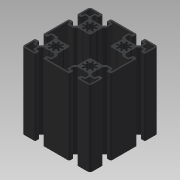
# Autodesk Inventor part: 45-9090
Saved by Autodesk Inventor 2013 (Build 170138000, 138)
## iProperties
Company: 80/20 Inc.
Created: 2014-04-23
Part Number: 45-9090
Material: Generic
Document SubType Name: Modeling
Designer: Ross Bowman
Density: 1 g/cm^3
Engineer: Ross Bowman
Catalog Web Link: 8020.net
Vendor: 80/20 Inc.
Material: 6105-T5 Aluminum
Author: Ross Bowman
Keywords: 80/20 , 8020 , T-Slot , Extrusion
Autodesk Inventor part; units mm, degrees
ref_plane "YZ Plane" through (0, 0, 0) normal (1, 0, 0) x (0, 1, 0)
ref_plane "XZ Plane" through (0, 0, 0) normal (0, 1, 0) x (-1, 0, 0)
ref_plane "XY Plane" through (0, 0, 0) normal (0, 0, 1) x (1, 0, 0)
sketch "Sketch1" plane through (0, 0, 0) normal (0, 0, 1) x (1, 0, 0)
  arc A0 (-37.7086, -41.7083) -> (-39.157, -41.2762) centre (-38.62, -42.1198) ccw
  arc A1 (-37.5167, -42.1716) -> (-37.7086, -41.7083) centre (-45, -45) ccw
  arc A2 (-38.2355, -43.5014) -> (-37.5167, -42.1716) centre (-38.4521, -42.5251) ccw
  line L0 (-38.2355, -43.5014) -> (-40.1182, -43.9192)
  arc A3 (-40.1181, -46.0805) -> (-40.1182, -43.9192) centre (-45, -45) ccw
  line L1 (-40.1181, -46.0805) -> (-38.2353, -46.4985)
  arc A4 (-37.5166, -47.8283) -> (-38.2353, -46.4985) centre (-38.452, -47.4747) ccw
  arc A5 (-37.7085, -48.2915) -> (-37.5166, -47.8283) centre (-45, -45) ccw
  arc A6 (-39.1571, -48.7236) -> (-37.7085, -48.2915) centre (-38.6199, -47.8801) ccw
  line L2 (-39.1571, -48.7236) -> (-40.7838, -47.6877)
  arc A7 (-42.312, -49.216) -> (-40.7838, -47.6877) centre (-45, -45) ccw
  line L3 (-42.312, -49.216) -> (-41.2762, -50.843)
  arc A8 (-41.7083, -52.2914) -> (-41.2762, -50.843) centre (-42.1198, -51.38) ccw
  arc A9 (-42.1716, -52.4833) -> (-41.7083, -52.2914) centre (-45, -45) ccw
  arc A10 (-43.5014, -51.7645) -> (-42.1716, -52.4833) centre (-42.5251, -51.5479) ccw
  line L4 (-43.5014, -51.7645) -> (-43.9192, -49.8818)
  arc A11 (-46.0805, -49.8819) -> (-43.9192, -49.8818) centre (-45, -45) ccw
  line L5 (-46.0805, -49.8819) -> (-46.4985, -51.7647)
  arc A12 (-47.8283, -52.4834) -> (-46.4985, -51.7647) centre (-47.4747, -51.548) ccw
  arc A13 (-48.2915, -52.2915) -> (-47.8283, -52.4834) centre (-45, -45) ccw
  arc A14 (-48.7236, -50.8429) -> (-48.2915, -52.2915) centre (-47.8801, -51.3801) ccw
  line L6 (-48.7236, -50.8429) -> (-47.6877, -49.2162)
  arc A15 (-49.216, -47.688) -> (-47.6877, -49.2162) centre (-45, -45) ccw
  line L7 (-49.216, -47.688) -> (-50.843, -48.7238)
  arc A16 (-52.2914, -48.2917) -> (-50.843, -48.7238) centre (-51.38, -47.8802) ccw
  arc A17 (-52.4833, -47.8284) -> (-52.2914, -48.2917) centre (-45, -45) ccw
  arc A18 (-51.7645, -46.4986) -> (-52.4833, -47.8284) centre (-51.5479, -47.4749) ccw
  line L8 (-51.7645, -46.4986) -> (-49.8818, -46.0808)
  arc A19 (-49.8819, -43.9195) -> (-49.8818, -46.0808) centre (-45, -45) ccw
  line L9 (-49.8819, -43.9195) -> (-51.7647, -43.5015)
  arc A20 (-52.4834, -42.1717) -> (-51.7647, -43.5015) centre (-51.548, -42.5253) ccw
  arc A21 (-52.2915, -41.7085) -> (-52.4834, -42.1717) centre (-45, -45) ccw
  arc A22 (-50.8429, -41.2764) -> (-52.2915, -41.7085) centre (-51.3801, -42.1199) ccw
  line L10 (-50.8429, -41.2764) -> (-49.2162, -42.3123)
  arc A23 (-47.688, -40.784) -> (-49.2162, -42.3123) centre (-45, -45) ccw
  line L11 (-47.688, -40.784) -> (-48.7238, -39.157)
  arc A24 (-48.2917, -37.7086) -> (-48.7238, -39.157) centre (-47.8802, -38.62) ccw
  arc A25 (-47.8284, -37.5167) -> (-48.2917, -37.7086) centre (-45, -45) ccw
  arc A26 (-46.4986, -38.2355) -> (-47.8284, -37.5167) centre (-47.4749, -38.4521) ccw
  line L12 (-46.4986, -38.2355) -> (-46.0808, -40.1182)
  arc A27 (-43.9195, -40.1181) -> (-46.0808, -40.1182) centre (-45, -45) ccw
  line L13 (-43.9195, -40.1181) -> (-43.5015, -38.2353)
  arc A28 (-42.1717, -37.5166) -> (-43.5015, -38.2353) centre (-42.5253, -38.452) ccw
  arc A29 (-41.7085, -37.7085) -> (-42.1717, -37.5166) centre (-45, -45) ccw
  arc A30 (-41.2764, -39.1571) -> (-41.7085, -37.7085) centre (-42.1199, -38.6199) ccw
  line L14 (-41.2764, -39.1571) -> (-42.3123, -40.7838)
  arc A31 (-40.784, -42.312) -> (-42.3123, -40.7838) centre (-45, -45) ccw
  line L15 (-40.784, -42.312) -> (-39.157, -41.2762)
  arc A32 (2.688, -49.216) -> (4.2162, -47.6877) centre (0, -45) ccw
  line L16 (2.688, -49.216) -> (3.7238, -50.843)
  arc A33 (3.2917, -52.2914) -> (3.7238, -50.843) centre (2.8802, -51.38) ccw
  arc A34 (2.8284, -52.4833) -> (3.2917, -52.2914) centre (0, -45) ccw
  arc A35 (1.4986, -51.7645) -> (2.8284, -52.4833) centre (2.4749, -51.5479) ccw
  line L17 (1.4986, -51.7645) -> (1.0808, -49.8818)
  arc A36 (-1.0805, -49.8819) -> (1.0808, -49.8818) centre (0, -45) ccw
  line L18 (-1.0805, -49.8819) -> (-1.4985, -51.7647)
  arc A37 (-2.8283, -52.4834) -> (-1.4985, -51.7647) centre (-2.4747, -51.548) ccw
  arc A38 (-3.2915, -52.2915) -> (-2.8283, -52.4834) centre (0, -45) ccw
  arc A39 (-3.7236, -50.8429) -> (-3.2915, -52.2915) centre (-2.8801, -51.3801) ccw
  line L19 (-3.7236, -50.8429) -> (-2.6877, -49.2162)
  arc A40 (-4.216, -47.688) -> (-2.6877, -49.2162) centre (0, -45) ccw
  line L20 (-4.216, -47.688) -> (-5.843, -48.7238)
  arc A41 (-7.2914, -48.2917) -> (-5.843, -48.7238) centre (-6.38, -47.8802) ccw
  arc A42 (-7.4833, -47.8284) -> (-7.2914, -48.2917) centre (0, -45) ccw
  arc A43 (-6.7645, -46.4986) -> (-7.4833, -47.8284) centre (-6.5479, -47.4749) ccw
  line L21 (-6.7645, -46.4986) -> (-4.8818, -46.0808)
  arc A44 (-4.8819, -43.9195) -> (-4.8818, -46.0808) centre (0, -45) ccw
  line L22 (-4.8819, -43.9195) -> (-6.7647, -43.5015)
  arc A45 (-7.4834, -42.1717) -> (-6.7647, -43.5015) centre (-6.548, -42.5253) ccw
  arc A46 (-7.2915, -41.7085) -> (-7.4834, -42.1717) centre (0, -45) ccw
  arc A47 (-5.8429, -41.2764) -> (-7.2915, -41.7085) centre (-6.3801, -42.1199) ccw
  line L23 (-5.8429, -41.2764) -> (-4.2162, -42.3123)
  arc A48 (-2.688, -40.784) -> (-4.2162, -42.3123) centre (0, -45) ccw
  line L24 (-2.688, -40.784) -> (-3.7238, -39.157)
  arc A49 (-3.2917, -37.7086) -> (-3.7238, -39.157) centre (-2.8802, -38.62) ccw
  arc A50 (-2.8284, -37.5167) -> (-3.2917, -37.7086) centre (0, -45) ccw
  arc A51 (-1.4986, -38.2355) -> (-2.8284, -37.5167) centre (-2.4749, -38.4521) ccw
  line L25 (-1.4986, -38.2355) -> (-1.0808, -40.1182)
  arc A52 (1.0805, -40.1181) -> (-1.0808, -40.1182) centre (0, -45) ccw
  line L26 (1.0805, -40.1181) -> (1.4985, -38.2353)
  arc A53 (2.8283, -37.5166) -> (1.4985, -38.2353) centre (2.4747, -38.452) ccw
  arc A54 (3.2915, -37.7085) -> (2.8283, -37.5166) centre (0, -45) ccw
  arc A55 (3.7236, -39.1571) -> (3.2915, -37.7085) centre (2.8801, -38.6199) ccw
  line L27 (3.7236, -39.1571) -> (2.6877, -40.7838)
  arc A56 (4.216, -42.312) -> (2.6877, -40.7838) centre (0, -45) ccw
  line L28 (4.216, -42.312) -> (5.843, -41.2762)
  arc A57 (7.2914, -41.7083) -> (5.843, -41.2762) centre (6.38, -42.1198) ccw
  arc A58 (7.4833, -42.1716) -> (7.2914, -41.7083) centre (0, -45) ccw
  arc A59 (6.7645, -43.5014) -> (7.4833, -42.1716) centre (6.5479, -42.5251) ccw
  line L29 (6.7645, -43.5014) -> (4.8818, -43.9192)
  arc A60 (4.8819, -46.0805) -> (4.8818, -43.9192) centre (0, -45) ccw
  line L30 (4.8819, -46.0805) -> (6.7647, -46.4985)
  arc A61 (7.4834, -47.8283) -> (6.7647, -46.4985) centre (6.548, -47.4747) ccw
  arc A62 (7.2915, -48.2915) -> (7.4834, -47.8283) centre (0, -45) ccw
  arc A63 (5.8429, -48.7236) -> (7.2915, -48.2915) centre (6.3801, -47.8801) ccw
  line L31 (5.8429, -48.7236) -> (4.2162, -47.6877)
  arc A64 (2.688, -4.216) -> (4.2162, -2.6877) centre (0, 0) ccw
  line L32 (2.688, -4.216) -> (3.7238, -5.843)
  arc A65 (3.2917, -7.2914) -> (3.7238, -5.843) centre (2.8802, -6.38) ccw
  arc A66 (2.8284, -7.4833) -> (3.2917, -7.2914) centre (0, 0) ccw
  arc A67 (1.4986, -6.7645) -> (2.8284, -7.4833) centre (2.4749, -6.5479) ccw
  line L33 (1.4986, -6.7645) -> (1.0808, -4.8818)
  arc A68 (-1.0805, -4.8819) -> (1.0808, -4.8818) centre (0, 0) ccw
  line L34 (-1.0805, -4.8819) -> (-1.4985, -6.7647)
  arc A69 (-2.8283, -7.4834) -> (-1.4985, -6.7647) centre (-2.4747, -6.548) ccw
  arc A70 (-3.2915, -7.2915) -> (-2.8283, -7.4834) centre (0, 0) ccw
  arc A71 (-3.7236, -5.8429) -> (-3.2915, -7.2915) centre (-2.8801, -6.3801) ccw
  line L35 (-3.7236, -5.8429) -> (-2.6877, -4.2162)
  arc A72 (-4.216, -2.688) -> (-2.6877, -4.2162) centre (0, 0) ccw
  line L36 (-4.216, -2.688) -> (-5.843, -3.7238)
  arc A73 (-7.2914, -3.2917) -> (-5.843, -3.7238) centre (-6.38, -2.8802) ccw
  arc A74 (-7.4833, -2.8284) -> (-7.2914, -3.2917) centre (0, 0) ccw
  arc A75 (-6.7645, -1.4986) -> (-7.4833, -2.8284) centre (-6.5479, -2.4749) ccw
  line L37 (-6.7645, -1.4986) -> (-4.8818, -1.0808)
  arc A76 (-4.8819, 1.0805) -> (-4.8818, -1.0808) centre (0, 0) ccw
  line L38 (-4.8819, 1.0805) -> (-6.7647, 1.4985)
  arc A77 (-7.4834, 2.8283) -> (-6.7647, 1.4985) centre (-6.548, 2.4747) ccw
  arc A78 (-7.2915, 3.2915) -> (-7.4834, 2.8283) centre (0, 0) ccw
  arc A79 (-5.8429, 3.7236) -> (-7.2915, 3.2915) centre (-6.3801, 2.8801) ccw
  line L39 (-5.8429, 3.7236) -> (-4.2162, 2.6877)
  arc A80 (-2.688, 4.216) -> (-4.2162, 2.6877) centre (0, 0) ccw
  line L40 (-2.688, 4.216) -> (-3.7238, 5.843)
  arc A81 (-3.2917, 7.2914) -> (-3.7238, 5.843) centre (-2.8802, 6.38) ccw
  arc A82 (-2.8284, 7.4833) -> (-3.2917, 7.2914) centre (0, 0) ccw
  arc A83 (-1.4986, 6.7645) -> (-2.8284, 7.4833) centre (-2.4749, 6.5479) ccw
  line L41 (-1.4986, 6.7645) -> (-1.0808, 4.8818)
  arc A84 (1.0805, 4.8819) -> (-1.0808, 4.8818) centre (0, 0) ccw
  line L42 (1.0805, 4.8819) -> (1.4985, 6.7647)
  arc A85 (2.8283, 7.4834) -> (1.4985, 6.7647) centre (2.4747, 6.548) ccw
  arc A86 (3.2915, 7.2915) -> (2.8283, 7.4834) centre (0, 0) ccw
  arc A87 (3.7236, 5.8429) -> (3.2915, 7.2915) centre (2.8801, 6.3801) ccw
  line L43 (3.7236, 5.8429) -> (2.6877, 4.2162)
  arc A88 (4.216, 2.688) -> (2.6877, 4.2162) centre (0, 0) ccw
  line L44 (4.216, 2.688) -> (5.843, 3.7238)
  arc A89 (7.2914, 3.2917) -> (5.843, 3.7238) centre (6.38, 2.8802) ccw
  arc A90 (7.4833, 2.8284) -> (7.2914, 3.2917) centre (0, 0) ccw
  arc A91 (6.7645, 1.4986) -> (7.4833, 2.8284) centre (6.5479, 2.4749) ccw
  line L45 (6.7645, 1.4986) -> (4.8818, 1.0808)
  arc A92 (4.8819, -1.0805) -> (4.8818, 1.0808) centre (0, 0) ccw
  line L46 (4.8819, -1.0805) -> (6.7647, -1.4985)
  arc A93 (7.4834, -2.8283) -> (6.7647, -1.4985) centre (6.548, -2.4747) ccw
  arc A94 (7.2915, -3.2915) -> (7.4834, -2.8283) centre (0, 0) ccw
  arc A95 (5.8429, -3.7236) -> (7.2915, -3.2915) centre (6.3801, -2.8801) ccw
  line L47 (5.8429, -3.7236) -> (4.2162, -2.6877)
  arc A96 (-37.7086, 3.2917) -> (-39.157, 3.7238) centre (-38.62, 2.8802) ccw
  arc A97 (-37.5167, 2.8284) -> (-37.7086, 3.2917) centre (-45, 0) ccw
  arc A98 (-38.2355, 1.4986) -> (-37.5167, 2.8284) centre (-38.4521, 2.4749) ccw
  line L48 (-38.2355, 1.4986) -> (-40.1182, 1.0808)
  arc A99 (-40.1181, -1.0805) -> (-40.1182, 1.0808) centre (-45, 0) ccw
  line L49 (-40.1181, -1.0805) -> (-38.2353, -1.4985)
  arc A100 (-37.5166, -2.8283) -> (-38.2353, -1.4985) centre (-38.452, -2.4747) ccw
  arc A101 (-37.7085, -3.2915) -> (-37.5166, -2.8283) centre (-45, 0) ccw
  arc A102 (-39.1571, -3.7236) -> (-37.7085, -3.2915) centre (-38.6199, -2.8801) ccw
  line L50 (-39.1571, -3.7236) -> (-40.7838, -2.6877)
  arc A103 (-42.312, -4.216) -> (-40.7838, -2.6877) centre (-45, 0) ccw
  line L51 (-42.312, -4.216) -> (-41.2762, -5.843)
  arc A104 (-41.7083, -7.2914) -> (-41.2762, -5.843) centre (-42.1198, -6.38) ccw
  arc A105 (-42.1716, -7.4833) -> (-41.7083, -7.2914) centre (-45, 0) ccw
  arc A106 (-43.5014, -6.7645) -> (-42.1716, -7.4833) centre (-42.5251, -6.5479) ccw
  line L52 (-43.5014, -6.7645) -> (-43.9192, -4.8818)
  arc A107 (-46.0805, -4.8819) -> (-43.9192, -4.8818) centre (-45, 0) ccw
  line L53 (-46.0805, -4.8819) -> (-46.4985, -6.7647)
  arc A108 (-47.8283, -7.4834) -> (-46.4985, -6.7647) centre (-47.4747, -6.548) ccw
  arc A109 (-48.2915, -7.2915) -> (-47.8283, -7.4834) centre (-45, 0) ccw
  arc A110 (-48.7236, -5.8429) -> (-48.2915, -7.2915) centre (-47.8801, -6.3801) ccw
  line L54 (-48.7236, -5.8429) -> (-47.6877, -4.2162)
  arc A111 (-49.216, -2.688) -> (-47.6877, -4.2162) centre (-45, 0) ccw
  line L55 (-49.216, -2.688) -> (-50.843, -3.7238)
  arc A112 (-52.2914, -3.2917) -> (-50.843, -3.7238) centre (-51.38, -2.8802) ccw
  arc A113 (-52.4833, -2.8284) -> (-52.2914, -3.2917) centre (-45, 0) ccw
  arc A114 (-51.7645, -1.4986) -> (-52.4833, -2.8284) centre (-51.5479, -2.4749) ccw
  line L56 (-51.7645, -1.4986) -> (-49.8818, -1.0808)
  arc A115 (-49.8819, 1.0805) -> (-49.8818, -1.0808) centre (-45, 0) ccw
  line L57 (-49.8819, 1.0805) -> (-51.7647, 1.4985)
  arc A116 (-52.4834, 2.8283) -> (-51.7647, 1.4985) centre (-51.548, 2.4747) ccw
  arc A117 (-52.2915, 3.2915) -> (-52.4834, 2.8283) centre (-45, 0) ccw
  arc A118 (-50.8429, 3.7236) -> (-52.2915, 3.2915) centre (-51.3801, 2.8801) ccw
  line L58 (-50.8429, 3.7236) -> (-49.2162, 2.6877)
  arc A119 (-47.688, 4.216) -> (-49.2162, 2.6877) centre (-45, 0) ccw
  line L59 (-47.688, 4.216) -> (-48.7238, 5.843)
  arc A120 (-48.2917, 7.2914) -> (-48.7238, 5.843) centre (-47.8802, 6.38) ccw
  arc A121 (-47.8284, 7.4833) -> (-48.2917, 7.2914) centre (-45, 0) ccw
  arc A122 (-46.4986, 6.7645) -> (-47.8284, 7.4833) centre (-47.4749, 6.5479) ccw
  line L60 (-46.4986, 6.7645) -> (-46.0808, 4.8818)
  arc A123 (-43.9195, 4.8819) -> (-46.0808, 4.8818) centre (-45, 0) ccw
  line L61 (-43.9195, 4.8819) -> (-43.5015, 6.7647)
  arc A124 (-42.1717, 7.4834) -> (-43.5015, 6.7647) centre (-42.5253, 6.548) ccw
  arc A125 (-41.7085, 7.2915) -> (-42.1717, 7.4834) centre (-45, 0) ccw
  arc A126 (-41.2764, 5.8429) -> (-41.7085, 7.2915) centre (-42.1199, 6.3801) ccw
  line L62 (-41.2764, 5.8429) -> (-42.3123, 4.2162)
  arc A127 (-40.784, 2.688) -> (-42.3123, 4.2162) centre (-45, 0) ccw
  line L63 (-40.784, 2.688) -> (-39.157, 3.7238)
  arc A128 (22.5, -6.585) -> (20.98, -5.065) centre (20.98, -6.585) ccw
  line L64 (18.02, -5.065) -> (20.98, -5.065)
  arc A129 (18.02, -5.065) -> (16.5, -6.585) centre (18.02, -6.585) ccw
  line L65 (16.5, -9.05) -> (16.5, -6.585)
  arc A130 (15.5, -10.05) -> (16.5, -9.05) centre (15.5, -9.05) ccw
  line L66 (12.4984, -10.05) -> (15.5, -10.05)
  arc A131 (12.2297, -9.9387) -> (12.4984, -10.05) centre (12.4984, -9.67) ccw
  line L67 (9.6113, -7.3203) -> (12.2297, -9.9387)
  arc A132 (9.5, -7.0516) -> (9.6113, -7.3203) centre (9.88, -7.0516) ccw
  line L68 (9.5, -0.9) -> (9.5, -7.0516)
  line L69 (8.9804, 0) -> (9.5, -0.9)
  line L70 (9.5, 0.9) -> (8.9804, 0)
  line L71 (9.5, 7.0516) -> (9.5, 0.9)
  arc A133 (9.6113, 7.3203) -> (9.5, 7.0516) centre (9.88, 7.0516) ccw
  line L72 (12.2297, 9.9387) -> (9.6113, 7.3203)
  arc A134 (12.4984, 10.05) -> (12.2297, 9.9387) centre (12.4984, 9.67) ccw
  line L73 (15.5, 10.05) -> (12.4984, 10.05)
  arc A135 (16.5, 9.05) -> (15.5, 10.05) centre (15.5, 9.05) ccw
  line L74 (16.5, 6.585) -> (16.5, 9.05)
  arc A136 (16.5, 6.585) -> (18.02, 5.065) centre (18.02, 6.585) ccw
  line L75 (20.98, 5.065) -> (18.02, 5.065)
  arc A137 (20.98, 5.065) -> (22.5, 6.585) centre (20.98, 6.585) ccw
  line L76 (22.5, 19.5) -> (22.5, 6.585)
  arc A138 (22.5, 19.5) -> (19.5, 22.5) centre (19.5, 19.5) ccw
  line L77 (6.585, 22.5) -> (19.5, 22.5)
  arc A139 (6.585, 22.5) -> (5.065, 20.98) centre (6.585, 20.98) ccw
  line L78 (5.065, 18.02) -> (5.065, 20.98)
  arc A140 (5.065, 18.02) -> (6.585, 16.5) centre (6.585, 18.02) ccw
  line L79 (9.05, 16.5) -> (6.585, 16.5)
  arc A141 (10.05, 15.5) -> (9.05, 16.5) centre (9.05, 15.5) ccw
  line L80 (10.05, 12.4984) -> (10.05, 15.5)
  arc A142 (9.9387, 12.2297) -> (10.05, 12.4984) centre (9.67, 12.4984) ccw
  line L81 (7.3203, 9.6113) -> (9.9387, 12.2297)
  arc A143 (7.0516, 9.5) -> (7.3203, 9.6113) centre (7.0516, 9.88) ccw
  line L82 (0.9, 9.5) -> (7.0516, 9.5)
  line L83 (0, 8.9849) -> (0.9, 9.5)
  line L84 (-0.9, 9.5) -> (0, 8.9849)
  line L85 (-7.0516, 9.5) -> (-0.9, 9.5)
  arc A144 (-7.3203, 9.6113) -> (-7.0516, 9.5) centre (-7.0516, 9.88) ccw
  line L86 (-9.9387, 12.2297) -> (-7.3203, 9.6113)
  arc A145 (-10.05, 12.4984) -> (-9.9387, 12.2297) centre (-9.67, 12.4984) ccw
  line L87 (-10.05, 15.5) -> (-10.05, 12.4984)
  arc A146 (-9.05, 16.5) -> (-10.05, 15.5) centre (-9.05, 15.5) ccw
  line L88 (-6.585, 16.5) -> (-9.05, 16.5)
  arc A147 (-6.585, 16.5) -> (-5.065, 18.02) centre (-6.585, 18.02) ccw
  line L89 (-5.065, 20.98) -> (-5.065, 18.02)
  arc A148 (-5.065, 20.98) -> (-6.585, 22.5) centre (-6.585, 20.98) ccw
  line L90 (-38.415, 22.5) -> (-6.585, 22.5)
  arc A149 (-38.415, 22.5) -> (-39.935, 20.98) centre (-38.415, 20.98) ccw
  line L91 (-39.935, 18.02) -> (-39.935, 20.98)
  arc A150 (-39.935, 18.02) -> (-38.415, 16.5) centre (-38.415, 18.02) ccw
  line L92 (-35.95, 16.5) -> (-38.415, 16.5)
  arc A151 (-34.95, 15.5) -> (-35.95, 16.5) centre (-35.95, 15.5) ccw
  line L93 (-34.95, 12.4984) -> (-34.95, 15.5)
  arc A152 (-35.0613, 12.2297) -> (-34.95, 12.4984) centre (-35.33, 12.4984) ccw
  line L94 (-37.6797, 9.6113) -> (-35.0613, 12.2297)
  arc A153 (-37.9484, 9.5) -> (-37.6797, 9.6113) centre (-37.9484, 9.88) ccw
  line L95 (-44.1, 9.5) -> (-37.9484, 9.5)
  line L96 (-45, 8.9849) -> (-44.1, 9.5)
  line L97 (-45.9, 9.5) -> (-45, 8.9849)
  line L98 (-52.0516, 9.5) -> (-45.9, 9.5)
  arc A154 (-52.3203, 9.6113) -> (-52.0516, 9.5) centre (-52.0516, 9.88) ccw
  line L99 (-54.9387, 12.2297) -> (-52.3203, 9.6113)
  arc A155 (-55.05, 12.4984) -> (-54.9387, 12.2297) centre (-54.67, 12.4984) ccw
  line L100 (-55.05, 15.5) -> (-55.05, 12.4984)
  arc A156 (-54.05, 16.5) -> (-55.05, 15.5) centre (-54.05, 15.5) ccw
  line L101 (-51.585, 16.5) -> (-54.05, 16.5)
  arc A157 (-51.585, 16.5) -> (-50.065, 18.02) centre (-51.585, 18.02) ccw
  line L102 (-50.065, 20.98) -> (-50.065, 18.02)
  arc A158 (-50.065, 20.98) -> (-51.585, 22.5) centre (-51.585, 20.98) ccw
  line L103 (-64.5, 22.5) -> (-51.585, 22.5)
  arc A159 (-64.5, 22.5) -> (-67.5, 19.5) centre (-64.5, 19.5) ccw
  line L104 (-67.5, 6.585) -> (-67.5, 19.5)
  arc A160 (-67.5, 6.585) -> (-65.98, 5.065) centre (-65.98, 6.585) ccw
  line L105 (-63.02, 5.065) -> (-65.98, 5.065)
  arc A161 (-63.02, 5.065) -> (-61.5, 6.585) centre (-63.02, 6.585) ccw
  line L106 (-61.5, 9.05) -> (-61.5, 6.585)
  arc A162 (-60.5, 10.05) -> (-61.5, 9.05) centre (-60.5, 9.05) ccw
  line L107 (-57.4984, 10.05) -> (-60.5, 10.05)
  arc A163 (-57.2297, 9.9387) -> (-57.4984, 10.05) centre (-57.4984, 9.67) ccw
  line L108 (-54.6113, 7.3203) -> (-57.2297, 9.9387)
  arc A164 (-54.5, 7.0516) -> (-54.6113, 7.3203) centre (-54.88, 7.0516) ccw
  line L109 (-54.5, 0.9) -> (-54.5, 7.0516)
  line L110 (-53.9804, 0) -> (-54.5, 0.9)
  line L111 (-54.5, -0.9) -> (-53.9804, 0)
  line L112 (-54.5, -7.0516) -> (-54.5, -0.9)
  arc A165 (-54.6113, -7.3203) -> (-54.5, -7.0516) centre (-54.88, -7.0516) ccw
  line L113 (-57.2297, -9.9387) -> (-54.6113, -7.3203)
  arc A166 (-57.4984, -10.05) -> (-57.2297, -9.9387) centre (-57.4984, -9.67) ccw
  line L114 (-60.5, -10.05) -> (-57.4984, -10.05)
  arc A167 (-61.5, -9.05) -> (-60.5, -10.05) centre (-60.5, -9.05) ccw
  line L115 (-61.5, -6.585) -> (-61.5, -9.05)
  arc A168 (-61.5, -6.585) -> (-63.02, -5.065) centre (-63.02, -6.585) ccw
  line L116 (-65.98, -5.065) -> (-63.02, -5.065)
  arc A169 (-65.98, -5.065) -> (-67.5, -6.585) centre (-65.98, -6.585) ccw
  line L117 (-67.5, -38.415) -> (-67.5, -6.585)
  arc A170 (-67.5, -38.415) -> (-65.98, -39.935) centre (-65.98, -38.415) ccw
  line L118 (-63.02, -39.935) -> (-65.98, -39.935)
  arc A171 (-63.02, -39.935) -> (-61.5, -38.415) centre (-63.02, -38.415) ccw
  line L119 (-61.5, -35.95) -> (-61.5, -38.415)
  arc A172 (-60.5, -34.95) -> (-61.5, -35.95) centre (-60.5, -35.95) ccw
  line L120 (-57.4984, -34.95) -> (-60.5, -34.95)
  arc A173 (-57.2297, -35.0613) -> (-57.4984, -34.95) centre (-57.4984, -35.33) ccw
  line L121 (-54.6113, -37.6797) -> (-57.2297, -35.0613)
  arc A174 (-54.5, -37.9484) -> (-54.6113, -37.6797) centre (-54.88, -37.9484) ccw
  line L122 (-54.5, -44.1) -> (-54.5, -37.9484)
  line L123 (-53.9804, -45) -> (-54.5, -44.1)
  line L124 (-54.5, -45.9) -> (-53.9804, -45)
  line L125 (-54.5, -52.0516) -> (-54.5, -45.9)
  arc A175 (-54.6113, -52.3203) -> (-54.5, -52.0516) centre (-54.88, -52.0516) ccw
  line L126 (-57.2297, -54.9387) -> (-54.6113, -52.3203)
  arc A176 (-57.4984, -55.05) -> (-57.2297, -54.9387) centre (-57.4984, -54.67) ccw
  line L127 (-60.5, -55.05) -> (-57.4984, -55.05)
  arc A177 (-61.5, -54.05) -> (-60.5, -55.05) centre (-60.5, -54.05) ccw
  line L128 (-61.5, -51.585) -> (-61.5, -54.05)
  arc A178 (-61.5, -51.585) -> (-63.02, -50.065) centre (-63.02, -51.585) ccw
  line L129 (-65.98, -50.065) -> (-63.02, -50.065)
  arc A179 (-65.98, -50.065) -> (-67.5, -51.585) centre (-65.98, -51.585) ccw
  line L130 (-67.5, -64.5) -> (-67.5, -51.585)
  arc A180 (-67.5, -64.5) -> (-64.5, -67.5) centre (-64.5, -64.5) ccw
  line L131 (-51.585, -67.5) -> (-64.5, -67.5)
  arc A181 (-51.585, -67.5) -> (-50.065, -65.98) centre (-51.585, -65.98) ccw
  line L132 (-50.065, -63.02) -> (-50.065, -65.98)
  arc A182 (-50.065, -63.02) -> (-51.585, -61.5) centre (-51.585, -63.02) ccw
  line L133 (-54.05, -61.5) -> (-51.585, -61.5)
  arc A183 (-55.05, -60.5) -> (-54.05, -61.5) centre (-54.05, -60.5) ccw
  line L134 (-55.05, -57.4984) -> (-55.05, -60.5)
  arc A184 (-54.9387, -57.2297) -> (-55.05, -57.4984) centre (-54.67, -57.4984) ccw
  line L135 (-52.3203, -54.6113) -> (-54.9387, -57.2297)
  arc A185 (-52.0516, -54.5) -> (-52.3203, -54.6113) centre (-52.0516, -54.88) ccw
  line L136 (-45.9, -54.5) -> (-52.0516, -54.5)
  line L137 (-45, -53.9849) -> (-45.9, -54.5)
  line L138 (-44.1, -54.5) -> (-45, -53.9849)
  line L139 (-37.9484, -54.5) -> (-44.1, -54.5)
  arc A186 (-37.6797, -54.6113) -> (-37.9484, -54.5) centre (-37.9484, -54.88) ccw
  line L140 (-35.0613, -57.2297) -> (-37.6797, -54.6113)
  arc A187 (-34.95, -57.4984) -> (-35.0613, -57.2297) centre (-35.33, -57.4984) ccw
  line L141 (-34.95, -60.5) -> (-34.95, -57.4984)
  arc A188 (-35.95, -61.5) -> (-34.95, -60.5) centre (-35.95, -60.5) ccw
  line L142 (-38.415, -61.5) -> (-35.95, -61.5)
  arc A189 (-38.415, -61.5) -> (-39.935, -63.02) centre (-38.415, -63.02) ccw
  line L143 (-39.935, -65.98) -> (-39.935, -63.02)
  arc A190 (-39.935, -65.98) -> (-38.415, -67.5) centre (-38.415, -65.98) ccw
  line L144 (-6.585, -67.5) -> (-38.415, -67.5)
  arc A191 (-6.585, -67.5) -> (-5.065, -65.98) centre (-6.585, -65.98) ccw
  line L145 (-5.065, -63.02) -> (-5.065, -65.98)
  arc A192 (-5.065, -63.02) -> (-6.585, -61.5) centre (-6.585, -63.02) ccw
  line L146 (-9.05, -61.5) -> (-6.585, -61.5)
  arc A193 (-10.05, -60.5) -> (-9.05, -61.5) centre (-9.05, -60.5) ccw
  line L147 (-10.05, -57.4984) -> (-10.05, -60.5)
  arc A194 (-9.9387, -57.2297) -> (-10.05, -57.4984) centre (-9.67, -57.4984) ccw
  line L148 (-7.3203, -54.6113) -> (-9.9387, -57.2297)
  arc A195 (-7.0516, -54.5) -> (-7.3203, -54.6113) centre (-7.0516, -54.88) ccw
  line L149 (-0.9, -54.5) -> (-7.0516, -54.5)
  line L150 (0, -53.9849) -> (-0.9, -54.5)
  line L151 (0.9, -54.5) -> (0, -53.9849)
  line L152 (7.0516, -54.5) -> (0.9, -54.5)
  arc A196 (7.3203, -54.6113) -> (7.0516, -54.5) centre (7.0516, -54.88) ccw
  line L153 (9.9387, -57.2297) -> (7.3203, -54.6113)
  arc A197 (10.05, -57.4984) -> (9.9387, -57.2297) centre (9.67, -57.4984) ccw
  line L154 (10.05, -60.5) -> (10.05, -57.4984)
  arc A198 (9.05, -61.5) -> (10.05, -60.5) centre (9.05, -60.5) ccw
  line L155 (6.585, -61.5) -> (9.05, -61.5)
  arc A199 (6.585, -61.5) -> (5.065, -63.02) centre (6.585, -63.02) ccw
  line L156 (5.065, -65.98) -> (5.065, -63.02)
  arc A200 (5.065, -65.98) -> (6.585, -67.5) centre (6.585, -65.98) ccw
  line L157 (19.5, -67.5) -> (6.585, -67.5)
  arc A201 (19.5, -67.5) -> (22.5, -64.5) centre (19.5, -64.5) ccw
  line L158 (22.5, -51.585) -> (22.5, -64.5)
  arc A202 (22.5, -51.585) -> (20.98, -50.065) centre (20.98, -51.585) ccw
  line L159 (18.02, -50.065) -> (20.98, -50.065)
  arc A203 (18.02, -50.065) -> (16.5, -51.585) centre (18.02, -51.585) ccw
  line L160 (16.5, -54.05) -> (16.5, -51.585)
  arc A204 (15.5, -55.05) -> (16.5, -54.05) centre (15.5, -54.05) ccw
  line L161 (12.4984, -55.05) -> (15.5, -55.05)
  arc A205 (12.2297, -54.9387) -> (12.4984, -55.05) centre (12.4984, -54.67) ccw
  line L162 (9.6113, -52.3203) -> (12.2297, -54.9387)
  arc A206 (9.5, -52.0516) -> (9.6113, -52.3203) centre (9.88, -52.0516) ccw
  line L163 (9.5, -45.9) -> (9.5, -52.0516)
  line L164 (8.9804, -45) -> (9.5, -45.9)
  line L165 (9.5, -44.1) -> (8.9804, -45)
  line L166 (9.5, -37.9484) -> (9.5, -44.1)
  arc A207 (9.6113, -37.6797) -> (9.5, -37.9484) centre (9.88, -37.9484) ccw
  line L167 (12.2297, -35.0613) -> (9.6113, -37.6797)
  arc A208 (12.4984, -34.95) -> (12.2297, -35.0613) centre (12.4984, -35.33) ccw
  line L168 (15.5, -34.95) -> (12.4984, -34.95)
  arc A209 (16.5, -35.95) -> (15.5, -34.95) centre (15.5, -35.95) ccw
  line L169 (16.5, -38.415) -> (16.5, -35.95)
  arc A210 (16.5, -38.415) -> (18.02, -39.935) centre (18.02, -38.415) ccw
  line L170 (20.98, -39.935) -> (18.02, -39.935)
  arc A211 (20.98, -39.935) -> (22.5, -38.415) centre (20.98, -38.415) ccw
  line L171 (22.5, -6.585) -> (22.5, -38.415)
  arc A212 (-56, 18.5) -> (-57, 17.5) centre (-56, 17.5) ccw
  line L172 (-57, 17.5) -> (-57, 12.38)
  arc A213 (-57.38, 12) -> (-57, 12.38) centre (-57.38, 12.38) ccw
  line L173 (-57.38, 12) -> (-62.5, 12)
  arc A214 (-62.5, 12) -> (-63.5, 11) centre (-62.5, 11) ccw
  line L174 (-63.5, 11) -> (-63.5, 9)
  arc A215 (-65.5, 9) -> (-63.5, 9) centre (-64.5, 9) ccw
  line L175 (-65.5, 9) -> (-65.5, 19.5)
  arc A216 (-64.5, 20.5) -> (-65.5, 19.5) centre (-64.5, 19.5) ccw
  line L176 (-64.5, 20.5) -> (-54, 20.5)
  arc A217 (-54, 18.5) -> (-54, 20.5) centre (-54, 19.5) ccw
  line L177 (-54, 18.5) -> (-56, 18.5)
  arc A218 (18.5, 11) -> (17.5, 12) centre (17.5, 11) ccw
  line L178 (17.5, 12) -> (12.38, 12)
  arc A219 (12, 12.38) -> (12.38, 12) centre (12.38, 12.38) ccw
  line L179 (12, 12.38) -> (12, 17.5)
  arc A220 (12, 17.5) -> (11, 18.5) centre (11, 17.5) ccw
  line L180 (11, 18.5) -> (9, 18.5)
  arc A221 (9, 20.5) -> (9, 18.5) centre (9, 19.5) ccw
  line L181 (9, 20.5) -> (19.5, 20.5)
  arc A222 (20.5, 19.5) -> (19.5, 20.5) centre (19.5, 19.5) ccw
  line L182 (20.5, 19.5) -> (20.5, 9)
  arc A223 (18.5, 9) -> (20.5, 9) centre (19.5, 9) ccw
  line L183 (18.5, 9) -> (18.5, 11)
  arc A224 (12.38, -57) -> (12, -57.38) centre (12.38, -57.38) ccw
  line L184 (12.38, -57) -> (17.5, -57)
  arc A225 (17.5, -57) -> (18.5, -56) centre (17.5, -56) ccw
  line L185 (18.5, -56) -> (18.5, -54)
  arc A226 (20.5, -54) -> (18.5, -54) centre (19.5, -54) ccw
  line L186 (20.5, -54) -> (20.5, -64.5)
  arc A227 (19.5, -65.5) -> (20.5, -64.5) centre (19.5, -64.5) ccw
  line L187 (19.5, -65.5) -> (9, -65.5)
  arc A228 (9, -63.5) -> (9, -65.5) centre (9, -64.5) ccw
  line L188 (9, -63.5) -> (11, -63.5)
  arc A229 (11, -63.5) -> (12, -62.5) centre (11, -62.5) ccw
  line L189 (12, -62.5) -> (12, -57.38)
  arc A230 (-63.5, -56) -> (-62.5, -57) centre (-62.5, -56) ccw
  line L190 (-62.5, -57) -> (-57.38, -57)
  arc A231 (-57, -57.38) -> (-57.38, -57) centre (-57.38, -57.38) ccw
  line L191 (-57, -57.38) -> (-57, -62.5)
  arc A232 (-57, -62.5) -> (-56, -63.5) centre (-56, -62.5) ccw
  line L192 (-56, -63.5) -> (-54, -63.5)
  arc A233 (-54, -65.5) -> (-54, -63.5) centre (-54, -64.5) ccw
  line L193 (-54, -65.5) -> (-64.5, -65.5)
  arc A234 (-65.5, -64.5) -> (-64.5, -65.5) centre (-64.5, -64.5) ccw
  line L194 (-65.5, -64.5) -> (-65.5, -54)
  arc A235 (-63.5, -54) -> (-65.5, -54) centre (-64.5, -54) ccw
  line L195 (-63.5, -54) -> (-63.5, -56)
  arc A236 (16.5, -12.34) -> (18.5, -10.34) centre (16.5, -10.34) ccw
  line L196 (18.5, -10.34) -> (18.5, -9)
  arc A237 (20.5, -9) -> (18.5, -9) centre (19.5, -9) ccw
  line L197 (20.5, -9) -> (20.5, -36)
  arc A238 (18.5, -36) -> (20.5, -36) centre (19.5, -36) ccw
  line L198 (18.5, -36) -> (18.5, -34.6651)
  arc A239 (18.5, -34.6651) -> (16.5, -32.6651) centre (16.5, -34.6651) ccw
  line L199 (16.5, -32.6651) -> (10.8723, -32.6651)
  arc A240 (10.8723, -32.6651) -> (9.4581, -33.2509) centre (10.8723, -34.6651) ccw
  line L200 (9.4581, -33.2509) -> (7.3203, -35.3887)
  arc A241 (7.0516, -35.5) -> (7.3203, -35.3887) centre (7.0516, -35.12) ccw
  line L201 (7.0516, -35.5) -> (0.9, -35.5)
  line L202 (0.9, -35.5) -> (0, -36.0151)
  line L203 (0, -36.0151) -> (-0.9, -35.5)
  line L204 (-0.9, -35.5) -> (-7.5, -35.5)
  arc A242 (-7.5, -35.5) -> (-9.5, -37.5) centre (-7.5, -37.5) ccw
  line L205 (-9.5, -37.5) -> (-9.5, -44.1)
  line L206 (-9.5, -44.1) -> (-8.9804, -45)
  line L207 (-8.9804, -45) -> (-9.5, -45.9)
  line L208 (-9.5, -45.9) -> (-9.5, -52.0516)
  arc A243 (-9.6113, -52.3203) -> (-9.5, -52.0516) centre (-9.88, -52.0516) ccw
  line L209 (-9.6113, -52.3203) -> (-11.1213, -53.8303)
  arc A244 (-11.1213, -53.8303) -> (-12, -55.9516) centre (-9, -55.9516) ccw
  line L210 (-12, -55.9516) -> (-12, -62.5)
  arc A245 (-12, -62.5) -> (-11, -63.5) centre (-11, -62.5) ccw
  line L211 (-11, -63.5) -> (-9, -63.5)
  arc A246 (-9, -65.5) -> (-9, -63.5) centre (-9, -64.5) ccw
  line L212 (-9, -65.5) -> (-36, -65.5)
  arc A247 (-36, -63.5) -> (-36, -65.5) centre (-36, -64.5) ccw
  line L213 (-36, -63.5) -> (-34, -63.5)
  arc A248 (-34, -63.5) -> (-33, -62.5) centre (-34, -62.5) ccw
  line L214 (-33, -62.5) -> (-33, -55.9516)
  arc A249 (-33, -55.9516) -> (-33.8787, -53.8303) centre (-36, -55.9516) ccw
  line L215 (-33.8787, -53.8303) -> (-35.3887, -52.3203)
  arc A250 (-35.5, -52.0516) -> (-35.3887, -52.3203) centre (-35.12, -52.0516) ccw
  line L216 (-35.5, -52.0516) -> (-35.5, -45.9)
  line L217 (-35.5, -45.9) -> (-36.0196, -45)
  line L218 (-36.0196, -45) -> (-35.5, -44.1)
  line L219 (-35.5, -44.1) -> (-35.5, -37.5)
  arc A251 (-35.5, -37.5) -> (-37.5, -35.5) centre (-37.5, -37.5) ccw
  line L220 (-37.5, -35.5) -> (-44.1, -35.5)
  line L221 (-44.1, -35.5) -> (-45, -36.0151)
  line L222 (-45, -36.0151) -> (-45.9, -35.5)
  line L223 (-45.9, -35.5) -> (-52.0516, -35.5)
  arc A252 (-52.3203, -35.3887) -> (-52.0516, -35.5) centre (-52.0516, -35.12) ccw
  line L224 (-52.3203, -35.3887) -> (-54.4632, -33.2458)
  arc A253 (-54.4632, -33.2458) -> (-55.8774, -32.66) centre (-55.8774, -34.66) ccw
  line L225 (-55.8774, -32.66) -> (-61.5, -32.66)
  arc A254 (-61.5, -32.66) -> (-63.5, -34.66) centre (-61.5, -34.66) ccw
  line L226 (-63.5, -34.66) -> (-63.5, -36)
  arc A255 (-65.5, -36) -> (-63.5, -36) centre (-64.5, -36) ccw
  line L227 (-65.5, -36) -> (-65.5, -9)
  arc A256 (-63.5, -9) -> (-65.5, -9) centre (-64.5, -9) ccw
  line L228 (-63.5, -9) -> (-63.5, -10.34)
  arc A257 (-63.5, -10.34) -> (-61.5, -12.34) centre (-61.5, -10.34) ccw
  line L229 (-61.5, -12.34) -> (-55.8774, -12.34)
  arc A258 (-55.8774, -12.34) -> (-54.4632, -11.7542) centre (-55.8774, -10.34) ccw
  line L230 (-54.4632, -11.7542) -> (-52.3203, -9.6113)
  arc A259 (-52.0516, -9.5) -> (-52.3203, -9.6113) centre (-52.0516, -9.88) ccw
  line L231 (-52.0516, -9.5) -> (-45.9, -9.5)
  line L232 (-45.9, -9.5) -> (-45, -8.9849)
  line L233 (-45, -8.9849) -> (-44.1, -9.5)
  line L234 (-44.1, -9.5) -> (-37.5, -9.5)
  arc A260 (-37.5, -9.5) -> (-35.5, -7.5) centre (-37.5, -7.5) ccw
  line L235 (-35.5, -7.5) -> (-35.5, -0.9)
  line L236 (-35.5, -0.9) -> (-36.0196, 0)
  line L237 (-36.0196, 0) -> (-35.5, 0.9)
  line L238 (-35.5, 0.9) -> (-35.5, 7.0516)
  arc A261 (-35.3887, 7.3203) -> (-35.5, 7.0516) centre (-35.12, 7.0516) ccw
  line L239 (-35.3887, 7.3203) -> (-33.8787, 8.8303)
  arc A262 (-33.8787, 8.8303) -> (-33, 10.9516) centre (-36, 10.9516) ccw
  line L240 (-33, 10.9516) -> (-33, 17.5)
  arc A263 (-33, 17.5) -> (-34, 18.5) centre (-34, 17.5) ccw
  line L241 (-34, 18.5) -> (-36, 18.5)
  arc A264 (-36, 20.5) -> (-36, 18.5) centre (-36, 19.5) ccw
  line L242 (-36, 20.5) -> (-9, 20.5)
  arc A265 (-9, 18.5) -> (-9, 20.5) centre (-9, 19.5) ccw
  line L243 (-9, 18.5) -> (-11, 18.5)
  arc A266 (-11, 18.5) -> (-12, 17.5) centre (-11, 17.5) ccw
  line L244 (-12, 17.5) -> (-12, 10.9516)
  arc A267 (-12, 10.9516) -> (-11.1213, 8.8303) centre (-9, 10.9516) ccw
  line L245 (-11.1213, 8.8303) -> (-9.6113, 7.3203)
  arc A268 (-9.5, 7.0516) -> (-9.6113, 7.3203) centre (-9.88, 7.0516) ccw
  line L246 (-9.5, 7.0516) -> (-9.5, 0.9)
  line L247 (-9.5, 0.9) -> (-8.9804, 0)
  line L248 (-8.9804, 0) -> (-9.5, -0.9)
  line L249 (-9.5, -0.9) -> (-9.5, -7.5)
  arc A269 (-9.5, -7.5) -> (-7.5, -9.5) centre (-7.5, -7.5) ccw
  line L250 (-7.5, -9.5) -> (-0.9, -9.5)
  line L251 (-0.9, -9.5) -> (0, -8.9849)
  line L252 (0, -8.9849) -> (0.9, -9.5)
  line L253 (0.9, -9.5) -> (7.0516, -9.5)
  arc A270 (7.3203, -9.6113) -> (7.0516, -9.5) centre (7.0516, -9.88) ccw
  line L254 (7.3203, -9.6113) -> (9.4632, -11.7542)
  arc A271 (9.4632, -11.7542) -> (10.8774, -12.34) centre (10.8774, -10.34) ccw
  line L255 (10.8774, -12.34) -> (16.5, -12.34)
  constraints: 544 point on circle, 512 end point, 272 centre point
extrude "Extrusion1" add sketch "Sketch1" against normal blind 100
body "Solid1"
